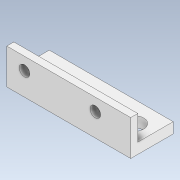
# Autodesk Inventor part: end_button
Saved by Autodesk Inventor 2022 (Build 260153000, 153)
## iProperties
Created: 2022-05-08
Part Number: end_button
Material: Generic
Document SubType Name: Modeling
Designer: ferna
Density: 1 g/cm^3
Appearance: White
Author: ferna
Autodesk Inventor part; units mm, degrees
ref_plane "YZ Plane" through (0, 0, 0) normal (1, 0, 0) x (0, 1, 0)
ref_plane "XZ Plane" through (0, 0, 0) normal (0, 1, 0) x (-1, 0, 0)
ref_plane "XY Plane" through (0, 0, 0) normal (0, 0, 1) x (1, 0, 0)
sketch "Sketch1" plane through (0, 0, 0) normal (0, 1, 0) x (-1, 0, 0)
  circle A0 centre (30.1, 6) radius 2.1
  circle A1 centre (49.9, 6) radius 2.1
  line L0 (0, 0) -> (80, 0)
  line L1 (80, 0) -> (80, 12)
  line L2 (0, 12) -> (80, 12)
  line L3 (0, 0) -> (0, 12)
  line L4 (40, 12) -> (15, 12)
  line L5 (15, 12) -> (15, 0)
  line L6 (15, 0) -> (65, 0)
  line L7 (65, 0) -> (65, 12)
  circle A2 centre (49.9, 6) radius 2.75
  circle A3 centre (30.1, 6) radius 2.75
  dimension "d0" = 25
  dimension "d1" = 50
  dimension "d2" = 5.5
  dimension "d3" = 5.5
  constraints: 16 end point, 4 centre point, 4 point on line, 2 coincident, 2 perpendicular, 1 midpoint
  measures "d0" distance of L4.start L4.end
  measures "d1" distance of L5.end L6.end
  measures "d2" diameter of A2
  measures "d3" diameter of A3
extrude "Extrusion1" add sketch "Sketch1" along normal blind 3 contours L5 L2 L7 L0
sketch "Sketch2" plane through (0, 3, 0) normal (0, 1, 0) x (1, 0, 0)
  line L0 (-15, -12) -> (-15, 0) projected
  line L1 (-65, 0) -> (-65, -12) projected
  line L2 (-15, -12) -> (-65, -12)
  line L3 (-65, -12) -> (-65, -9.9998)
  line L4 (-65, -9.9998) -> (-15, -9.9998)
  line L5 (-15, -9.9998) -> (-15, -12)
  point P0 (0, 0)
  constraints: 8 end point, 2 parallel, 1 horizontal, 1 perpendicular, 1 point on line
extrude "Extrusion2" add sketch "Sketch2" along normal blind 7
sketch "Sketch3" plane through (-15, 3, 9.9998) normal (0, 0, -1) x (-1, 0, 0)
  line L0 (0, -3) -> (0, 7) projected
  line L1 (0, -0.0684) -> (30, -0.0684)
  line L2 (0, -0.0684) -> (30, -0.0684) construction
  line L3 (30, -0.0684) -> (30, 3.4316)
  line L4 (30, 3.4316) -> (40, 3.4316)
  line L5 (40, 3.4316) -> (20, 3.4316)
  circle A0 centre (20, 3.4316) radius 1.5
  circle A1 centre (40, 3.4316) radius 1.5
  point P0 (-15, -3)
  dimension "d8" = 30
  dimension "d9" = 0
  dimension "d10" = 3.5
  dimension "d11" = 10
  dimension "d12" = 20
  dimension "d13" = 3
  dimension "d14" = 3
  constraints: 10 end point, 3 perpendicular, 2 centre point, 2 coincident, 2 point on line, 1 collinear, 1 horizontal
  measures "d8" distance of L1.start L1.end
  measures "d9" distance between parallel lines of L1 L2
  measures "d10" distance of L1.end L3.end
  measures "d11" distance of L3.end L4.end
  measures "d12" distance of L4.end L5.end
  measures "d13" diameter of A0
  measures "d14" diameter of A1
extrude "Extrusion3" cut sketch "Sketch3" against normal blind 10
sketch "Sketch4" plane through (-15, 0, 12) normal (1, 0, 0) x (0, 0, -1)
  line L0 (0, 0) -> (12, 0) projected
  line L1 (12, 0) -> (12, 3) projected
  line L2 (2.0002, 3) -> (12, 3) projected
  line L3 (2.0002, 3) -> (2.0002, 10) projected
  line L4 (0, 10) -> (2.0002, 10) projected
  line L5 (0, 0) -> (0, 10) projected
extrude "Extrusion4" cut sketch "Sketch4" against normal blind 10
sketch "Sketch5" plane through (-65, 0, 0) normal (-1, 0, 0) x (0, 0, 1)
  line L0 (8.75, 3) -> (8.75, 0) projected
  line L1 (0, 0) -> (12, 0) projected
  line L2 (12, 0) -> (12, 10) projected
  line L3 (9.9998, 10) -> (12, 10) projected
  line L4 (9.9998, 3) -> (9.9998, 10) projected
  line L5 (0, 3) -> (9.9998, 3) projected
  line L6 (0, 0) -> (0, 3) projected
extrude "Extrusion5" cut sketch "Sketch5" against normal blind 5
body "Solid1"
